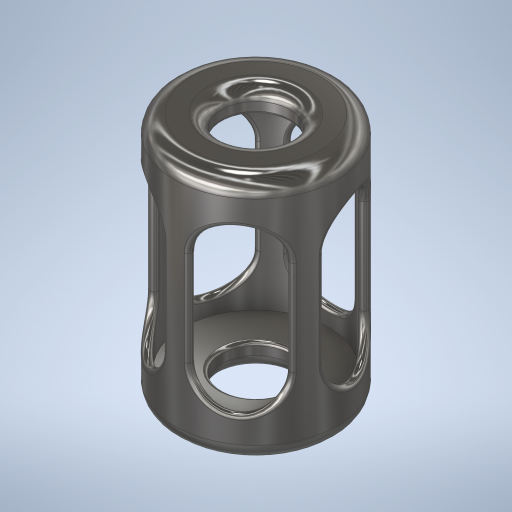
# Autodesk Inventor part: klec
Saved by Autodesk Inventor 2023 (Build 270158000, 158)
## iProperties
Created: 2024-01-16
Part Number: klec
Material: Všeobecné
Document SubType Name: Modeling
Designer: 42073
Density: 1 g/cm^3
Appearance: Ocel – leštěná
Mass: 29.2703 g
Surface Area: 158.415 cm^2
Volume: 29.2703 cm^3
Author: 42073
Autodesk Inventor part; units mm, degrees
ref_plane "YZ Plane" through (0, 0, 0) normal (1, 0, 0) x (0, 1, 0)
sketch "Náčrt1" plane through (0, 0, 0) normal (0, 0, 1) x (1, 0, 0)
  circle A0 centre (0, 0) radius 24
  dimension "d0" = 48
  constraints: 1 centre point, 1 coincident
  measures "d0" diameter of A0
extrude "Vysunutí1" add sketch "Náčrt1" along normal blind 73
sketch "Náčrt2" plane through (0, 0, 73) normal (0, 0, 1) x (1, 0, 0)
  circle A0 centre (0, 0) radius 10
  dimension "d3" = 20
  constraints: 1 centre point, 1 coincident
  measures "d3" diameter of A0
extrude "Vysunutí2" cut sketch "Náčrt2" against normal blind 73
ref_plane "Pracovní rovina1" through (0, 0, 7.5) normal (0, 0, -1) x (-1, 0, 0)
sketch "Náčrt3" plane through (0, 0, 7.5) normal (0, 0, -1) x (-1, 0, 0)
  circle A0 centre (0, 0) radius 21.5
  dimension "d7" = 43
  constraints: 1 centre point, 1 coincident
  measures "d7" diameter of A0
extrude "Vysunutí3" cut sketch "Náčrt3" against normal blind 58
fillet "Zaoblení1" radius 5 2 edges at (-24, 0, 73) (-24, 0, 0)
ref_plane "Pracovní rovina2" through (0, 24, 0) normal (0, 1, 0) x (-1, 0, 0)
sketch "Náčrt4" plane through (0, 24, 0) normal (0, 1, 0) x (-1, 0, 0)
  line L0 (-10, 50.5) -> (-10, 22.5)
  line L1 (0, 12.5) -> (0, 12.5)
  line L2 (10, 22.5) -> (10, 50.5)
  line L3 (0, 60.5) -> (0, 60.5)
  arc A0 (0, 60.5) -> (-10, 50.5) centre (0, 50.5) ccw
  arc A1 (10, 50.5) -> (0, 60.5) centre (0, 50.5) ccw
  arc A2 (0, 12.5) -> (10, 22.5) centre (0, 22.5) ccw
  arc A3 (-10, 22.5) -> (0, 12.5) centre (0, 22.5) ccw
  point P0 (0, 0)
  point P1 (-10, 60.5)
  point P2 (-10, 12.5)
  point P3 (10, 12.5)
  point P4 (10, 60.5)
  dimension "d15" = 48
  dimension "d16" = 20
  dimension "d17" = 48
  dimension "d18" = 10
  constraints: 8 end point, 8 point on circle, 8 point on line, 8 tangent, 4 centre point, 3 equal radius, 1 horizontal, 1 perpendicular
  measures "d15" distance of point (-10, 60.5) point (-10, 12.5)
  measures "d16" distance of point (-10, 12.5) point (10, 12.5)
  measures "d17" distance of point (10, 12.5) point (10, 60.5)
  measures "d18" radius of A0
extrude "Vysunutí4" cut sketch "Náčrt4" against normal blind 10
pattern_circular "Kruhové pole1" count 5 over 360 about axis through (0, 0, 73) along (0, 0, -1) of "Vysunutí4"
fillet "Zaoblení2" radius 4 2 edges at (-10, 0, 73) (-10, 0, 0)
fillet "Zaoblení3" radius 1 2 edges at (-10, 0, 7.5) (-10, 0, 65.5)
fillet "Zaoblení4" radius 1.25 20 edges at (16.7746, 13.4485, 56.9914) (21.1915, -3.6291, 36.5) (21.4758, -1.0202, 16.0086) (15.0112, 15.392, 36.5) (7.6067, 20.1094, 16.0086) (-10, 19.0329, 36.5) (-7.6067, 20.1094, 56.9914) (10, 19.0329, 36.5) (5.6661, -20.7399, 16.0086) (19.2774, -9.5201, 36.5) (17.974, -11.7977, 56.9914) (3.0971, -21.2758, 36.5) (-5.6661, -20.74, 56.9914) (-19.2774, -9.5201, 36.5) (-17.9739, -11.7978, 16.0086) (-3.0971, -21.2758, 36.5) (-16.7746, 13.4485, 16.0086) (-21.1915, -3.6291, 36.5) (-21.3282, -2.7128, 54.4871) (-15.0112, 15.392, 36.5)
fillet "Zaoblení5" radius 1.25 21 edges at (17.6594, 16.2525, 36.5) (23.7891, 3.1745, 13.4871) (23.9102, -2.0745, 18.9842) (23.8398, -2.7686, 36.5) (19.2963, 14.2707, 56.9883) (7.6093, 22.7618, 16.0116) (10, 21.8174, 36.5) (-7.6093, 22.7618, 56.9883) (-10, 21.8174, 36.5) (-17.6594, 16.2525, 36.5) (-23.9991, -0.2031, 56.9883) (-23.8398, -2.7686, 36.5) (-19.2964, 14.2706, 16.0116) (-20.9141, -11.7728, 36.5) (-7.223, -22.8873, 56.9883) (-4.7338, -23.5285, 36.5) (-19.5351, -13.9421, 16.0116) (7.223, -22.8873, 16.0116) (4.7338, -23.5285, 36.5) (19.5351, -13.942, 56.9883) (20.9141, -11.7728, 36.5)
